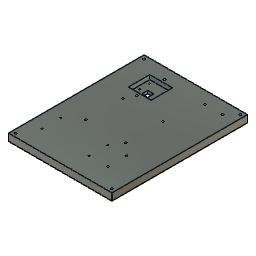
Platform1 (v2~recovered) (Autodesk Fusion 360 design; units mm, degrees)
Autodesk Fusion 360 part; units mm, degrees
form "Form1" [no effect] in component "Component"
sketch "sketch 245" plane through (0, 0, 0) normal (0, 0, 1) x (1, 0, 0)
  line L0 (0, 0) -> (145, 0)
  line L1 (145, 0) -> (145, 190)
  line L2 (145, 190) -> (0, 190)
  line L3 (0, 190) -> (0, 0)
  constraint horizontal L0
  constraint vertical L1
  constraint horizontal L2
  constraint vertical L3
  constraint coincident L0.start L3.end
extrude "Extrude1" add sketch "sketch 245" along normal blind 10 in component "Component"
sketch "Sketch1" plane through (0, 0, 10) normal (0, 0, 1) x (-1, 0, 0) in component "Component"
  line L0 (0, -190) -> (0, 0)
  line L1 (0, 0) -> (-145, 0)
  line L2 (-145, 0) -> (-145, -190)
  line L3 (-145, -190) -> (0, -190)
  line L4 (-28, -140) -> (-60, -140)
  line L5 (-60, -140) -> (-60, -170)
  line L6 (-60, -170) -> (-28, -170)
  line L7 (-28, -170) -> (-28, -140)
  dimension "d5" = 32
  dimension "d6" = 30
  constraint horizontal L4
  constraint vertical L5
  constraint horizontal L6
  constraint vertical L7
  measures "d5" distance of L4.start L4.end
  measures "d6" distance of L4.start L6.end
extrude "Extrude2" cut sketch "Sketch1" against normal blind 6 contours L4 L5 L6 L7 in component "Component"
sketch "Sketch2" plane through (0, 0, 10) normal (0, 0, 1) x (-1, 0, 0) in component "Component"
  line L0 (-60, -140) -> (-28, -140)
  line L1 (-28, -140) -> (-28, -170)
  line L2 (-28, -170) -> (-60, -170)
  line L3 (-60, -170) -> (-60, -140)
  line L4 (0, -190) -> (0, 0)
  line L5 (0, 0) -> (-145, 0)
  line L6 (-145, 0) -> (-145, -190)
  line L7 (-145, -190) -> (0, -190)
  line L8 (-39.7504, -148.5003) -> (-48.2504, -148.5003)
  line L9 (-48.2504, -148.5003) -> (-48.2504, -157.0003)
  line L10 (-48.2504, -157.0003) -> (-39.7504, -157.0003)
  line L11 (-39.7504, -157.0003) -> (-39.7504, -148.5003)
  dimension "d9" = 8.5
  dimension "d10" = 8.5
  constraint horizontal L8
  constraint vertical L9
  constraint horizontal L10
  constraint vertical L11
  measures "d9" distance of L8.start L8.end
  measures "d10" distance of L8.start L10.end
sketch "Sketch3" plane through (0, 0, 10) normal (0, 0, 1) x (-1, 0, 0) in component "Component"
  line L0 (-60, -140) -> (-28, -140)
  line L1 (-28, -140) -> (-28, -170)
  line L2 (-28, -170) -> (-60, -170)
  line L3 (-60, -170) -> (-60, -140)
  line L4 (0, -190) -> (0, 0)
  line L5 (0, 0) -> (-145, 0)
  line L6 (-145, 0) -> (-145, -190)
  line L7 (-145, -190) -> (0, -190)
  line L8 (-39.7504, -146.9997) -> (-48.2504, -146.9997)
  line L9 (-48.2504, -146.9997) -> (-48.2504, -155.4997)
  line L10 (-48.2504, -155.4997) -> (-39.7504, -155.4997)
  line L11 (-39.7504, -155.4997) -> (-39.7504, -146.9997)
  dimension "d11" = 8.5
  dimension "d12" = 8.5
  constraint horizontal L8
  constraint vertical L9
  constraint horizontal L10
  constraint vertical L11
  measures "d11" distance of L8.start L8.end
  measures "d12" distance of L8.start L10.end
extrude "Extrude3" cut sketch "Sketch3" against normal blind 10 contours L8 L9 L10 L11 in component "Component"
sketch "Sketch4" plane through (0, 0, 10) normal (0, 0, 1) x (-1, 0, 0) in component "Component"
  line L0 (-60, -140) -> (-28, -140)
  line L1 (-28, -140) -> (-28, -170)
  line L2 (-28, -170) -> (-60, -170)
  line L3 (-60, -170) -> (-60, -140)
  line L4 (0, -190) -> (0, 0)
  line L5 (0, 0) -> (-145, 0)
  line L6 (-145, 0) -> (-145, -190)
  line L7 (-145, -190) -> (0, -190)
  circle A0 centre (-44.25, -135.4997) radius 1.5
  dimension "d15" = 3
  measures "d15" diameter of A0
sketch "Sketch5" plane through (0, 0, 10) normal (0, 0, 1) x (-1, 0, 0) in component "Component"
  circle A0 centre (-44.2496, -174.5004) radius 1.5
  dimension "d18" = 3
  measures "d18" diameter of A0
extrude "Extrude5" cut sketch "Sketch4" against normal blind 8 contours A0 in component "Component"
extrude "Extrude6" cut sketch "Sketch5" against normal blind 8 in component "Component"
sketch "Sketch6" plane through (0, 0, 10) normal (0, 0, 1) x (-1, 0, 0) in component "Component"
  circle A0 centre (-110.2995, -54.9997) radius 1.5
  dimension "d23" = 3
  measures "d23" diameter of A0
extrude "Extrude7" cut sketch "Sketch6" against normal blind 8 in component "Component"
sketch "Sketch7" plane through (0, 0, 10) normal (0, 0, 1) x (-1, 0, 0) in component "Component"
  circle A0 centre (-110.3, -29) radius 1.5
  dimension "d26" = 3
  measures "d26" diameter of A0
extrude "Extrude8" cut sketch "Sketch7" against normal blind 8 in component "Component"
sketch "Sketch8" plane through (0, 0, 10) normal (0, 0, 1) x (-1, 0, 0) in component "Component"
  circle A0 centre (-102.9997, -172.5003) radius 1.5
  dimension "d29" = 3
  measures "d29" diameter of A0
extrude "Extrude9" cut sketch "Sketch8" against normal blind 0.8 in component "Component"
sketch "Sketch9" plane through (0, 0, 10) normal (0, 0, 1) x (-1, 0, 0) in component "Component"
  circle A0 centre (-127.5999, -172.4996) radius 1.5
  dimension "d32" = 3
  measures "d32" diameter of A0
extrude "Extrude10" cut sketch "Sketch9" against normal blind 0.8 in component "Component"
sketch "Sketch10" plane through (0, 0, 10) normal (0, 0, 1) x (-1, 0, 0) in component "Component"
  circle A0 centre (-38.0004, -122.5001) radius 1.5
  dimension "d35" = 3
  measures "d35" diameter of A0
extrude "Extrude11" cut sketch "Sketch10" against normal blind 0.8 in component "Component"
sketch "Sketch11" plane through (0, 0, 10) normal (0, 0, 1) x (-1, 0, 0) in component "Component"
  circle A0 centre (-38, -70.5) radius 1.5
  dimension "d38" = 3
  measures "d38" diameter of A0
extrude "Extrude12" cut sketch "Sketch11" against normal blind 0.8 in component "Component"
sketch "Sketch12" plane through (0, 0, 10) normal (0, 0, 1) x (-1, 0, 0) in component "Component"
  circle A0 centre (-94.0001, -122.5002) radius 1.5
  dimension "d42" = 3
  measures "d42" diameter of A0
extrude "Extrude13" cut sketch "Sketch12" against normal blind 0.8 in component "Component"
sketch "Sketch13" plane through (0, 0, 10) normal (0, 0, 1) x (-1, 0, 0) in component "Component"
  circle A0 centre (-94, -70.5) radius 1.5
  dimension "d45" = 3
  measures "d45" diameter of A0
extrude "Extrude14" cut sketch "Sketch13" against normal blind 0.8 in component "Component"
extrude "Extrude15" cut sketch "Sketch12" against normal blind 8 in component "Component"
extrude "Extrude16" cut sketch "Sketch10" against normal blind 8 in component "Component"
extrude "Extrude17" cut sketch "Sketch11" against normal blind 8 in component "Component"
extrude "Extrude18" cut sketch "Sketch13" against normal blind 8 in component "Component"
sketch "Sketch15" plane through (0, 0, 10) normal (0, 0, 1) x (-1, 0, 0) in component "Component"
  circle A0 centre (-94, -70.5) radius 1.5
  circle A1 centre (-94.0001, -122.5002) radius 1.5
  circle A2 centre (-38, -70.5) radius 1.5
  circle A3 centre (-38.0004, -122.5001) radius 1.5
  circle A4 centre (-127.5999, -172.4996) radius 1.5
  circle A5 centre (-102.9997, -172.5003) radius 1.5
  circle A6 centre (-110.3, -29) radius 1.5
  circle A7 centre (-110.2995, -54.9997) radius 1.5
  circle A8 centre (-44.2496, -174.5004) radius 1.5
  circle A9 centre (-44.25, -135.4997) radius 1.5
  line L0 (-60, -140) -> (-28, -140)
  line L1 (-28, -140) -> (-28, -170)
  line L2 (-28, -170) -> (-60, -170)
  line L3 (-60, -170) -> (-60, -140)
  line L4 (0, -190) -> (0, 0)
  line L5 (0, 0) -> (-145, 0)
  line L6 (-145, 0) -> (-145, -190)
  line L7 (-145, -190) -> (0, -190)
  circle A10 centre (-5, -5) radius 1.5
  dimension "d58" = 3
  measures "d58" diameter of A10
extrude "Extrude19" cut sketch "Sketch15" against normal blind 8 contours A10 in component "Component"
sketch "Sketch16" plane through (0, 0, 10) normal (0, 0, 1) x (-1, 0, 0) in component "Component"
  circle A0 centre (-5, -5) radius 1.5
  circle A1 centre (-94, -70.5) radius 1.5
  circle A2 centre (-94.0001, -122.5002) radius 1.5
  circle A3 centre (-38, -70.5) radius 1.5
  circle A4 centre (-38.0004, -122.5001) radius 1.5
  circle A5 centre (-127.5999, -172.4996) radius 1.5
  circle A6 centre (-102.9997, -172.5003) radius 1.5
  circle A7 centre (-110.3, -29) radius 1.5
  circle A8 centre (-110.2995, -54.9997) radius 1.5
  circle A9 centre (-44.2496, -174.5004) radius 1.5
  circle A10 centre (-44.25, -135.4997) radius 1.5
  line L0 (-60, -140) -> (-28, -140)
  line L1 (-28, -140) -> (-28, -170)
  line L2 (-28, -170) -> (-60, -170)
  line L3 (-60, -170) -> (-60, -140)
  line L4 (0, -190) -> (0, 0)
  line L5 (0, 0) -> (-145, 0)
  line L6 (-145, 0) -> (-145, -190)
  line L7 (-145, -190) -> (0, -190)
  circle A11 centre (-5, -185) radius 1.5
  dimension "d61" = 3
  measures "d61" diameter of A11
extrude "Extrude20" cut sketch "Sketch16" against normal blind 8 contours A11 in component "Component"
sketch "Sketch17" plane through (0, 0, 10) normal (0, 0, 1) x (-1, 0, 0) in component "Component"
  circle A0 centre (-5, -185) radius 1.5
  circle A1 centre (-5, -5) radius 1.5
  circle A2 centre (-94, -70.5) radius 1.5
  circle A3 centre (-94.0001, -122.5002) radius 1.5
  circle A4 centre (-38, -70.5) radius 1.5
  circle A5 centre (-38.0004, -122.5001) radius 1.5
  circle A6 centre (-127.5999, -172.4996) radius 1.5
  circle A7 centre (-102.9997, -172.5003) radius 1.5
  circle A8 centre (-110.3, -29) radius 1.5
  circle A9 centre (-110.2995, -54.9997) radius 1.5
  circle A10 centre (-44.2496, -174.5004) radius 1.5
  circle A11 centre (-44.25, -135.4997) radius 1.5
  line L0 (-60, -140) -> (-28, -140)
  line L1 (-28, -140) -> (-28, -170)
  line L2 (-28, -170) -> (-60, -170)
  line L3 (-60, -170) -> (-60, -140)
  line L4 (0, -190) -> (0, 0)
  line L5 (0, 0) -> (-145, 0)
  line L6 (-145, 0) -> (-145, -190)
  line L7 (-145, -190) -> (0, -190)
  circle A12 centre (-140, -5) radius 1.5
  dimension "d64" = 3
  measures "d64" diameter of A12
extrude "Extrude21" cut sketch "Sketch17" against normal blind 8 contours A12 in component "Component"
sketch "Sketch18" plane through (0, 0, 10) normal (0, 0, 1) x (-1, 0, 0) in component "Component"
  circle A0 centre (-140, -5) radius 1.5
  circle A1 centre (-5, -185) radius 1.5
  circle A2 centre (-5, -5) radius 1.5
  circle A3 centre (-94, -70.5) radius 1.5
  circle A4 centre (-94.0001, -122.5002) radius 1.5
  circle A5 centre (-38, -70.5) radius 1.5
  circle A6 centre (-38.0004, -122.5001) radius 1.5
  circle A7 centre (-127.5999, -172.4996) radius 1.5
  circle A8 centre (-102.9997, -172.5003) radius 1.5
  circle A9 centre (-110.3, -29) radius 1.5
  circle A10 centre (-110.2995, -54.9997) radius 1.5
  circle A11 centre (-44.2496, -174.5004) radius 1.5
  circle A12 centre (-44.25, -135.4997) radius 1.5
  line L0 (-60, -140) -> (-28, -140)
  line L1 (-28, -140) -> (-28, -170)
  line L2 (-28, -170) -> (-60, -170)
  line L3 (-60, -170) -> (-60, -140)
  line L4 (0, -190) -> (0, 0)
  line L5 (0, 0) -> (-145, 0)
  line L6 (-145, 0) -> (-145, -190)
  line L7 (-145, -190) -> (0, -190)
  circle A13 centre (-140, -185) radius 1.5
  dimension "d67" = 3
  measures "d67" diameter of A13
extrude "Extrude22" cut sketch "Sketch18" against normal blind 8 contours A13 in component "Component"
extrude "Extrude23" cut 1 faces at (102.688, 172.8912, 9.2) along direction (0, 0, -1) blind 8 in component "Component"
extrude "Extrude24" cut 1 faces at (127.6535, 172.1087, 9.2) along direction (0, 0, -1) blind 8 in component "Component"
sketch "Sketch19" plane through (0, 0, 10) normal (0, 0, 1) x (-1, 0, 0) in component "Component"
  circle A0 centre (-140, -185) radius 1.5
  circle A1 centre (-140, -5) radius 1.5
  circle A2 centre (-5, -185) radius 1.5
  circle A3 centre (-5, -5) radius 1.5
  circle A4 centre (-94, -70.5) radius 1.5
  circle A5 centre (-94.0001, -122.5002) radius 1.5
  circle A6 centre (-38, -70.5) radius 1.5
  circle A7 centre (-38.0004, -122.5001) radius 1.5
  circle A8 centre (-127.5999, -172.4996) radius 1.5
  circle A9 centre (-102.9997, -172.5003) radius 1.5
  circle A10 centre (-110.3, -29) radius 1.5
  circle A11 centre (-110.2995, -54.9997) radius 1.5
  circle A12 centre (-44.2496, -174.5004) radius 1.5
  circle A13 centre (-44.25, -135.4997) radius 1.5
  line L0 (-60, -140) -> (-28, -140)
  line L1 (-28, -140) -> (-28, -170)
  line L2 (-28, -170) -> (-60, -170)
  line L3 (-60, -170) -> (-60, -140)
  line L4 (0, -190) -> (0, 0)
  line L5 (0, 0) -> (-145, 0)
  line L6 (-145, 0) -> (-145, -190)
  line L7 (-145, -190) -> (0, -190)
  circle A14 centre (-18, -55) radius 1
  dimension "d74" = 2
  measures "d74" diameter of A14
extrude "Extrude25" cut sketch "Sketch19" against normal blind 8 contours A14 in component "Component"
sketch "Sketch20" plane through (0, 0, 10) normal (0, 0, 1) x (-1, 0, 0) in component "Component"
  circle A0 centre (-18, -55) radius 1
  circle A1 centre (-140, -185) radius 1.5
  circle A2 centre (-140, -5) radius 1.5
  circle A3 centre (-5, -185) radius 1.5
  circle A4 centre (-5, -5) radius 1.5
  circle A5 centre (-94, -70.5) radius 1.5
  circle A6 centre (-94.0001, -122.5002) radius 1.5
  circle A7 centre (-38, -70.5) radius 1.5
  circle A8 centre (-38.0004, -122.5001) radius 1.5
  circle A9 centre (-127.5999, -172.4996) radius 1.5
  circle A10 centre (-102.9997, -172.5003) radius 1.5
  circle A11 centre (-110.3, -29) radius 1.5
  circle A12 centre (-110.2995, -54.9997) radius 1.5
  circle A13 centre (-44.2496, -174.5004) radius 1.5
  circle A14 centre (-44.25, -135.4997) radius 1.5
  line L0 (-60, -140) -> (-28, -140)
  line L1 (-28, -140) -> (-28, -170)
  line L2 (-28, -170) -> (-60, -170)
  line L3 (-60, -170) -> (-60, -140)
  line L4 (0, -190) -> (0, 0)
  line L5 (0, 0) -> (-145, 0)
  line L6 (-145, 0) -> (-145, -190)
  line L7 (-145, -190) -> (0, -190)
  circle A15 centre (-18, -29) radius 1
  dimension "d77" = 2
  measures "d77" diameter of A15
extrude "Extrude26" cut sketch "Sketch20" against normal blind 8 contours A15 in component "Component"
sketch "Sketch21" plane through (0, 0, 10) normal (0, 0, 1) x (-1, 0, 0) in component "Component"
  circle A0 centre (-18, -29) radius 1
  circle A1 centre (-18, -55) radius 1
  circle A2 centre (-140, -185) radius 1.5
  circle A3 centre (-140, -5) radius 1.5
  circle A4 centre (-5, -185) radius 1.5
  circle A5 centre (-5, -5) radius 1.5
  circle A6 centre (-94, -70.5) radius 1.5
  circle A7 centre (-94.0001, -122.5002) radius 1.5
  circle A8 centre (-38, -70.5) radius 1.5
  circle A9 centre (-38.0004, -122.5001) radius 1.5
  circle A10 centre (-127.5999, -172.4996) radius 1.5
  circle A11 centre (-102.9997, -172.5003) radius 1.5
  circle A12 centre (-110.3, -29) radius 1.5
  circle A13 centre (-110.2995, -54.9997) radius 1.5
  circle A14 centre (-44.2496, -174.5004) radius 1.5
  circle A15 centre (-44.25, -135.4997) radius 1.5
  line L0 (-60, -140) -> (-28, -140)
  line L1 (-28, -140) -> (-28, -170)
  line L2 (-28, -170) -> (-60, -170)
  line L3 (-60, -170) -> (-60, -140)
  line L4 (0, -190) -> (0, 0)
  line L5 (0, 0) -> (-145, 0)
  line L6 (-145, 0) -> (-145, -190)
  line L7 (-145, -190) -> (0, -190)
  circle A16 centre (-84, -55) radius 1
  dimension "d80" = 2
  measures "d80" diameter of A16
extrude "Extrude27" cut sketch "Sketch21" against normal blind 8 contours A16 in component "Component"
sketch "Sketch22" plane through (0, 0, 10) normal (0, 0, 1) x (-1, 0, 0) in component "Component"
  circle A0 centre (-84, -55) radius 1
  circle A1 centre (-18, -29) radius 1
  circle A2 centre (-18, -55) radius 1
  circle A3 centre (-140, -185) radius 1.5
  circle A4 centre (-140, -5) radius 1.5
  circle A5 centre (-5, -185) radius 1.5
  circle A6 centre (-5, -5) radius 1.5
  circle A7 centre (-94, -70.5) radius 1.5
  circle A8 centre (-94.0001, -122.5002) radius 1.5
  circle A9 centre (-38, -70.5) radius 1.5
  circle A10 centre (-38.0004, -122.5001) radius 1.5
  circle A11 centre (-127.5999, -172.4996) radius 1.5
  circle A12 centre (-102.9997, -172.5003) radius 1.5
  circle A13 centre (-110.3, -29) radius 1.5
  circle A14 centre (-110.2995, -54.9997) radius 1.5
  circle A15 centre (-44.2496, -174.5004) radius 1.5
  circle A16 centre (-44.25, -135.4997) radius 1.5
  line L0 (-60, -140) -> (-28, -140)
  line L1 (-28, -140) -> (-28, -170)
  line L2 (-28, -170) -> (-60, -170)
  line L3 (-60, -170) -> (-60, -140)
  line L4 (0, -190) -> (0, 0)
  line L5 (0, 0) -> (-145, 0)
  line L6 (-145, 0) -> (-145, -190)
  line L7 (-145, -190) -> (0, -190)
  circle A17 centre (-84, -29) radius 1
  dimension "d83" = 2
  measures "d83" diameter of A17
extrude "Extrude28" cut sketch "Sketch22" against normal blind 8 contours A17 in component "Component"
sketch "Sketch23" plane through (0, 0, 10) normal (0, 0, 1) x (-1, 0, 0) in component "Component"
  circle A0 centre (-84, -29) radius 1
  circle A1 centre (-84, -55) radius 1
  circle A2 centre (-18, -29) radius 1
  circle A3 centre (-18, -55) radius 1
  circle A4 centre (-140, -185) radius 1.5
  circle A5 centre (-140, -5) radius 1.5
  circle A6 centre (-5, -185) radius 1.5
  circle A7 centre (-5, -5) radius 1.5
  circle A8 centre (-94, -70.5) radius 1.5
  circle A9 centre (-94.0001, -122.5002) radius 1.5
  circle A10 centre (-38, -70.5) radius 1.5
  circle A11 centre (-38.0004, -122.5001) radius 1.5
  circle A12 centre (-127.5999, -172.4996) radius 1.5
  circle A13 centre (-102.9997, -172.5003) radius 1.5
  circle A14 centre (-110.3, -29) radius 1.5
  circle A15 centre (-110.2995, -54.9997) radius 1.5
  circle A16 centre (-44.2496, -174.5004) radius 1.5
  circle A17 centre (-44.25, -135.4997) radius 1.5
  line L0 (-60, -140) -> (-28, -140)
  line L1 (-28, -140) -> (-28, -170)
  line L2 (-28, -170) -> (-60, -170)
  line L3 (-60, -170) -> (-60, -140)
  line L4 (0, -190) -> (0, 0)
  line L5 (0, 0) -> (-145, 0)
  line L6 (-145, 0) -> (-145, -190)
  line L7 (-145, -190) -> (0, -190)
sketch "Sketch24" plane through (0, 0, 10) normal (0, 0, 1) x (-1, 0, 0) in component "Component"
  circle A0 centre (-32.75, -164.75) radius 1
  dimension "d87" = 2
  measures "d87" diameter of A0
sketch "Sketch25" plane through (0, 0, 10) normal (0, 0, 1) x (-1, 0, 0) in component "Component"
  circle A0 centre (-32.75, -151.25) radius 1
  dimension "d88" = 2
  measures "d88" diameter of A0
sketch "Sketch26" plane through (0, 0, 10) normal (0, 0, 1) x (-1, 0, 0) in component "Component"
  circle A0 centre (-55.25, -151.25) radius 1
  dimension "d89" = 2
  measures "d89" diameter of A0
sketch "Sketch27" plane through (0, 0, 10) normal (0, 0, 1) x (-1, 0, 0) in component "Component"
  circle A0 centre (-55.25, -164.75) radius 1
  dimension "d90" = 2
  measures "d90" diameter of A0
extrude "Extrude29" cut sketch "Sketch24" against normal blind 10 in component "Component"
extrude "Extrude30" cut sketch "Sketch27" against normal blind 10 in component "Component"
extrude "Extrude31" cut sketch "Sketch26" against normal blind 10 in component "Component"
extrude "Extrude32" cut sketch "Sketch25" against normal blind 10 in component "Component"
extrude "Extrude4" [suppressed] in component "Component"
component "Component" placed x (1, 0, 0) y (0, 1, 0) z (0, 0, 1) at (0, 0, 0)
